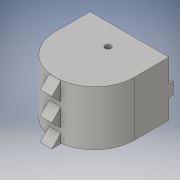
# Autodesk Inventor part: Skin1
Saved by Autodesk Inventor 2016 (Build 200138000, 138)
## iProperties
Created: 2017-03-07
Part Number: Skin1
Material: Generic
Document SubType Name: Modeling
Designer: Owner
Density: 1 g/cm^3
Appearance: Default
Author: Owner
Autodesk Inventor part; units mm, degrees
ref_plane "YZ Plane" through (0, 0, 0) normal (1, 0, 0) x (0, 1, 0)
ref_plane "XZ Plane" through (0, 0, 0) normal (0, 1, 0) x (-1, 0, 0)
ref_plane "XY Plane" through (0, 0, 0) normal (0, 0, 1) x (1, 0, 0)
sketch "Sketch1" plane through (0, 0, 0) normal (0, 0, 1) x (1, 0, 0)
  arc A0 (-38.1, -57.15) -> (38.1, -57.15) centre (0, -57.15) ccw projected
  line L0 (38.1, -57.15) -> (43.1, -57.15) projected
  line L1 (43.1, -57.15) -> (43.1, 62.15) projected
  line L2 (43.1, 62.15) -> (-43.1, 62.15) projected
  line L3 (-43.1, 62.15) -> (-43.1, -57.15) projected
  line L4 (-43.1, -57.15) -> (-38.1, -57.15) projected
  line L5 (14, 57.15) -> (-14, 57.15) projected
  line L6 (14, 57.15) -> (14, 54.15) projected
  line L7 (14, 54.15) -> (-10.002, 54.15) projected
  line L8 (-10.002, 54.15) -> (-10.002, 53.078) projected
  line L9 (-10.002, 53.078) -> (-14, 53.078) projected
  line L10 (-14, 53.078) -> (-14, 57.15) projected
  line L11 (10.16, -7.55) -> (-10.16, -7.55) projected
  line L12 (-10.16, -7.55) -> (-10.16, 9.15) projected
  line L13 (-10.16, 9.15) -> (10.16, 9.15) projected
  line L14 (10.16, 9.15) -> (10.16, -7.55) projected
  circle A1 centre (0, -77.15) radius 5 projected
  line L15 (-19.058, -20.782) -> (-19.058, -16.21) projected
  line L16 (-19.058, -16.21) -> (-17.058, -16.21) projected
  line L17 (-17.058, -16.21) -> (-17.058, -22.782) projected
  line L18 (-17.058, -22.782) -> (-24.598, -22.782) projected
  line L19 (-24.598, -22.782) -> (-24.598, -16.21) projected
  line L20 (-24.598, -16.21) -> (-22.598, -16.21) projected
  line L21 (-22.598, -16.21) -> (-22.598, -20.782) projected
  line L22 (-22.598, -20.782) -> (-19.058, -20.782) projected
  line L23 (-19.058, 7.65) -> (-19.058, 12.222) projected
  line L24 (-19.058, 12.222) -> (-22.598, 12.222) projected
  line L25 (-22.598, 12.222) -> (-22.598, 7.65) projected
  line L26 (-22.598, 7.65) -> (-24.598, 7.65) projected
  line L27 (-24.598, 7.65) -> (-24.598, 14.222) projected
  line L28 (-24.598, 14.222) -> (-17.058, 14.222) projected
  line L29 (-17.058, 14.222) -> (-17.058, 7.65) projected
  line L30 (-17.058, 7.65) -> (-19.058, 7.65) projected
  line L31 (-6.662, 29.218) -> (-6.662, 22.4) projected
  line L32 (-6.662, 22.4) -> (7.275, 22.4) projected
  line L33 (7.275, 22.4) -> (7.275, 19.4) projected
  line L34 (7.275, 19.4) -> (-14.202, 19.4) projected
  line L35 (-14.202, 19.4) -> (-14.202, 29.218) projected
  line L36 (-14.202, 29.218) -> (-12.202, 29.218) projected
  line L37 (-12.202, 29.218) -> (-12.202, 29.221) projected
  line L38 (-12.202, 29.221) -> (-8.662, 29.221) projected
  line L39 (-8.662, 29.221) -> (-8.662, 29.218) projected
  line L40 (-8.662, 29.218) -> (-6.662, 29.218) projected
  line L41 (38.1, -57.15) -> (43.1, -57.15)
  line L42 (43.1, -57.15) -> (43.1, 62.15)
  line L43 (43.1, 62.15) -> (38.1, 62.15)
  line L44 (38.1, 62.15) -> (38.1, -57.15)
  line L45 (-38.1, -57.15) -> (-43.1, -57.15)
  line L46 (-43.1, -57.15) -> (-43.1, 62.15)
  line L47 (-43.1, 62.15) -> (-38.1, 62.15)
  line L48 (-38.1, 62.15) -> (-38.1, -57.15)
  line L49 (-43.1, 62.15) -> (-43.1, 57.15)
  line L50 (-43.1, 57.15) -> (43.1, 57.15)
  line L51 (43.1, 57.15) -> (-43.1, 57.15)
  line L52 (-43.1, 57.15) -> (-43.1, 62.15)
  line L53 (-43.1, 62.15) -> (43.1, 62.15)
  line L54 (43.1, 62.15) -> (43.1, 57.15)
  point P0 (0, 0)
  dimension "d0" = 5
  constraints: 28 end point, 6 parallel, 4 perpendicular, 3 horizontal, 2 point on line
  measures "d0" distance of L2.end L49.end
extrude "Extrusion1" add sketch "Sketch1" along normal blind 38.1 contours L4 L3 L50 L48 | L44 L50 L1 L0 | L50 L3 L2 L48 | L48 L2 L44 L50 L5 | L44 L2 L1 L50
sketch "Sketch2" plane through (-43.1, -57.15, 0) normal (0, -1, 0) x (1, 0, 0)
  line L0 (5, 38.1) -> (81.2, 38.1) projected
  arc A0 (81.2, 38.1) -> (5, 38.1) centre (43.1, 38.1) ccw
  line L1 (0, 38.1) -> (5, 38.1) projected
  arc A1 (86.2, 38.1) -> (0, 38.1) centre (43.1, 38.1) ccw
  line L2 (0, 38.1) -> (5, 38.1)
  line L3 (81.2, 38.1) -> (86.2, 38.1) projected
  line L4 (81.2, 38.1) -> (86.2, 38.1)
  point P0 (43.1, 0)
  constraints: 4 end point, 4 point on circle, 2 centre point, 2 horizontal, 1 coincident, 1 midpoint
extrude "Extrusion2" add sketch "Sketch2" against normal blind 119.3 contours L1 A1 L3 A0
sketch "Sketch3" plane through (-43.1, 62.15, 0) normal (0, 1, 0) x (1, 0, 0)
  arc A0 (5, -38.1) -> (81.2, -38.1) centre (43.1, -38.1) ccw projected
  line L0 (81.2, -38.1) -> (5, -38.1) projected
  point P0 (43.1, 0)
extrude "Extrusion3" add sketch "Sketch3" against normal blind 5
sketch "Sketch4" plane through (-43.1, 62.15, 0) normal (0, 1, 0) x (1, 0, 0)
  circle A0 centre (43.1, -23.375) radius 3.275 projected
  point P0 (43.1, 0)
extrude "Extrusion4" cut sketch "Sketch4" against normal blind 5
ref_plane "Work Plane1" through (0.0038, -57.15, 0) normal (-1, 0, 0) x (0, 0, 1)
sketch "Sketch5" plane through (0.0038, -57.15, 0) normal (-1, 0, 0) x (0, 0, 1)
  point P0 (0, 57.15)
sketch "Sketch6" plane through (0.0038, -57.15, 0) normal (-1, 0, 0) x (0, 0, 1)
  line L0 (81.2, 0) -> (81.2, 119.3) projected
  line L1 (81.2, 119.3) -> (81.2, 99.3)
  line L2 (81.2, 109.3) -> (91.2, 109.3)
  line L3 (91.2, 109.3) -> (81.2, 119.3)
  line L4 (91.2, 109.3) -> (81.2, 99.3)
  line L5 (91.2, 84.475) -> (81.2, 74.475)
  line L6 (81.2, 84.475) -> (91.2, 84.475)
  line L7 (81.2, 94.475) -> (81.2, 74.475)
  line L8 (91.2, 84.475) -> (81.2, 94.475)
  line L9 (91.2, 59.65) -> (81.2, 49.65)
  line L10 (81.2, 59.65) -> (91.2, 59.65)
  line L11 (81.2, 69.65) -> (81.2, 49.65)
  line L12 (91.2, 59.65) -> (81.2, 69.65)
  line L13 (91.2, 34.825) -> (81.2, 24.825)
  line L14 (81.2, 34.825) -> (91.2, 34.825)
  line L15 (81.2, 44.825) -> (81.2, 24.825)
  line L16 (91.2, 34.825) -> (81.2, 44.825)
  line L17 (91.2, 10) -> (81.2, 0)
  line L18 (81.2, 10) -> (91.2, 10)
  line L19 (81.2, 20) -> (81.2, 0)
  line L20 (91.2, 10) -> (81.2, 20)
  point P0 (0, 57.15)
  dimension "d10" = 20
  dimension "d11" = 10
  dimension "d14" = 24.825
  constraints: 40 end point, 1 horizontal, 1 midpoint, 1 point on line, 1 vertical, 32 other
  measures "d10" distance of L0.end L1.end
  measures "d11" distance of L2.start L2.end
  measures "d14" distance of L2.end L5.start
extrude "Extrusion5" add sketch "Sketch6" along normal mid plane 12.7
sketch "Sketch8" plane through (0, 0, 0) normal (0, 0, -1) x (-1, 0, 0)
  line L0 (40.1, 24.05) -> (40.1, 36.75) projected
  line L1 (40.1, -31.75) -> (40.1, -19.05) projected
  line L2 (-40.1, 36.75) -> (-40.1, 24.05) projected
  line L3 (-40.1, -19.05) -> (-40.1, -31.75) projected
  line L4 (43.1, 62.15) -> (43.1, -57.15) projected
  line L5 (40.1, 36.75) -> (43.1, 36.75)
  line L6 (43.1, 36.75) -> (43.1, 24.05)
  line L7 (43.1, 24.05) -> (40.1, 24.05)
  line L8 (40.1, 24.05) -> (40.1, 36.75)
  line L9 (40.1, -19.05) -> (43.1, -19.05)
  line L10 (43.1, -19.05) -> (43.1, -31.75)
  line L11 (43.1, -31.75) -> (40.1, -31.75)
  line L12 (40.1, -31.75) -> (40.1, -19.05)
  line L13 (-43.1, -57.15) -> (-43.1, 62.15) projected
  line L14 (-40.1, -19.05) -> (-43.1, -19.05)
  line L15 (-43.1, -19.05) -> (-43.1, -31.75)
  line L16 (-43.1, -31.75) -> (-40.1, -31.75)
  line L17 (-40.1, -31.75) -> (-40.1, -19.05)
  line L18 (-40.1, 24.05) -> (-43.1, 24.05)
  line L19 (-43.1, 24.05) -> (-43.1, 36.75)
  line L20 (-43.1, 36.75) -> (-40.1, 36.75)
  line L21 (-40.1, 36.75) -> (-40.1, 24.05)
  point P0 (0, 0)
  constraints: 32 end point, 8 parallel, 6 point on line, 4 horizontal, 4 perpendicular
extrude "Extrusion6" add sketch "Sketch8" along normal blind 5.0038
sketch "Sketch9" plane through (43.1, -57.15, 38.1) normal (1, 0, 0) x (0, 0, -1)
  line L0 (-53.1, 59.65) -> (-43.1, 69.65) projected
  line L1 (-53.1, 59.65) -> (78.849, 59.65)
  line L2 (78.849, 59.65) -> (83.1956, -43.5453)
  line L3 (83.1956, -43.5453) -> (-80.8871, -47.5296)
  line L4 (-80.8871, -47.5296) -> (-53.1, 59.65)
  point P0 (38.1, 57.15)
  constraints: 8 end point, 1 horizontal
extrude "Extrusion7" cut sketch "Sketch9" against normal blind 2540
body "Solid1"
